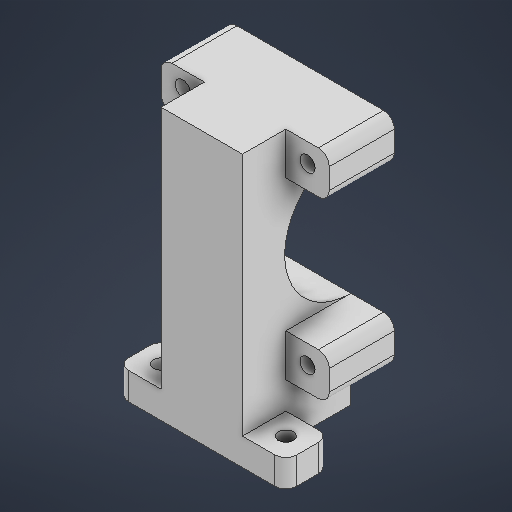
# Autodesk Inventor part: üst döner blok
Saved by Autodesk Inventor 2026.1 (Build 301233020, 233B)
## iProperties
Created: 2026-04-16
Part Number: üst döner blok
Material: Generic
Document SubType Name: Modeling
Designer: kadir
Density: 1 g/cm^3
Appearance: Default
Author: kadir
Autodesk Inventor part; units mm, degrees
ref_plane "YZ Plane" through (0, 0, 0) normal (1, 0, 0) x (0, 1, 0)
ref_plane "XZ Plane" through (0, 0, 0) normal (0, 1, 0) x (-1, 0, 0)
sketch "Sketch1" plane through (0, 0, 0) normal (0, 0, 1) x (1, 0, 0)
  line L0 (0, 0) -> (15, 0)
  line L1 (15, 0) -> (15, 50)
  line L2 (15, 50) -> (0, 50)
  line L3 (0, 50) -> (0, 0)
  dimension "d0" = 15
  dimension "d1" = 50
  constraints: 8 end point, 2 parallel, 1 horizontal, 1 perpendicular
  measures "d0" distance of L2.end L1.end
  measures "d1" distance of L1.end L0.end
extrude "Extrusion1" add sketch "Sketch1" along normal blind 20
sketch "Sketch2" plane through (15, 0, 0) normal (1, 0, 0) x (0, 0, -1)
  circle A0 centre (0, 30) radius 12.2
  line L0 (0, 50) -> (-20, 50) projected
  line L1 (0, 0) -> (0, 50) projected
  line L2 (0, 50) -> (0, 0)
  line L3 (-20, 0) -> (-20, 50) projected
  point P0 (0, 17.8)
  point P1 (0, 42.2)
  dimension "d4" = 24.4
  dimension "d5" = 20
  dimension "d6" = 20
  constraints: 2 end point, 1 centre point, 1 vertical
  measures "d4" diameter of A0
  measures "d5" distance from line of L0 A0.centre
  measures "d6" distance from line of L3 A0.centre
extrude "Extrusion2" cut sketch "Sketch2" against normal through all contours L1 A0 picked at (-4.6431, 33.0439)
sketch "Sketch3" plane through (15, 0, 20) normal (1, 0, 0) x (0, 0, -1)
  line L0 (20, 50) -> (0, 50) projected
  line L1 (20, 50) -> (8, 50)
  line L2 (8, 50) -> (8, 42.2)
  line L3 (8, 42.2) -> (20, 42.2)
  line L4 (20, 42.2) -> (20, 50)
  line L5 (-6.7049, 30) -> (32.7164, 30)
  line L6 (20, 10) -> (0, 10)
  line L7 (8, 10) -> (8, 17.8)
  line L8 (8, 17.8) -> (20, 17.8)
  line L9 (20, 17.8) -> (20, 10)
  point P0 (20, 0)
  dimension "d9" = 12
  dimension "d10" = 7.8
  dimension "d11" = 20
  constraints: 18 end point, 5 symmetric about line, 2 horizontal, 2 parallel, 1 perpendicular
  measures "d9" distance of L3.end L2.end
  measures "d10" distance of L2.end L1.end
  measures "d11" distance between parallel lines of L0 L5
extrude "Extrusion3" add sketch "Sketch3" along normal blind 8
sketch "Sketch4" plane through (0, 0, 0) normal (0, 0, -1) x (-1, 0, 0)
  circle A0 centre (-19, 46.5) radius 1.4
  line L0 (0, 50) -> (-23, 50) projected
  line L1 (-23, 42.2) -> (-23, 50) projected
  circle A1 centre (-19, 14.3) radius 1.4
  line L2 (-15, 17.8) -> (-23, 17.8) projected
  line L3 (-23, 10) -> (-23, 17.8) projected
  point P0 (0, 0)
  dimension "d14" = 2.8
  dimension "d15" = 3.5
  dimension "d16" = 4
  dimension "d17" = 2.8
  dimension "d18" = 3.5
  dimension "d43" = 4
  constraints: 2 centre point
  measures "d14" diameter of A0
  measures "d15" distance from line of L0 A0.centre
  measures "d16" distance from line of L1 A0.centre
  measures "d17" diameter of A1
  measures "d18" distance from line of L2 A1.centre
  measures "d43" distance from line of L3 A1.centre
extrude "Extrusion4" cut sketch "Sketch4" against normal through all
sketch "Sketch5" plane through (0, 0, 20) normal (-1, 0, 0) x (0, 0, 1)
  line L0 (-20, 42.2) -> (-20, 50) projected
  line L1 (-8, 42.2) -> (-20, 42.2) projected
  line L2 (-20, 50) -> (-8, 50)
  line L3 (-8, 50) -> (-8, 42.2)
  line L4 (-8, 42.2) -> (-20, 42.2)
  line L5 (-20, 42.2) -> (-20, 50)
  arc A0 (-20, 17.8) -> (-20, 42.2) centre (-20, 30) ccw projected
  line L6 (-8, 10) -> (-20, 10) projected
  line L7 (-20, 17.8) -> (-8, 17.8)
  line L8 (-8, 17.8) -> (-8, 10)
  line L9 (-8, 10) -> (-20, 10)
  line L10 (-20, 10) -> (-20, 17.8)
  point P0 (-20, 0)
  constraints: 16 end point, 4 parallel, 2 horizontal, 2 perpendicular
extrude "Extrusion5" add sketch "Sketch5" along normal blind 8
sketch "Sketch6" plane through (0, 0, 0) normal (0, 0, -1) x (-1, 0, 0)
  circle A0 centre (4, 47) radius 1.4
  line L0 (8, 50) -> (8, 42.2) projected
  line L1 (8, 50) -> (-23, 50) projected
  circle A1 centre (4, 14.8) radius 1.4
  line L2 (0, 17.8) -> (8, 17.8) projected
  line L3 (8, 17.8) -> (8, 10) projected
  point P0 (0, 0)
  point P1 (8, 46.1)
  dimension "d23" = 2.8
  dimension "d24" = 4
  dimension "d25" = 3
  dimension "d26" = 2.8
  dimension "d27" = 3
  dimension "d44" = 4
  constraints: 2 centre point, 1 midpoint
  measures "d23" diameter of A0
  measures "d24" horizontal distance of point (8, 46.1) A0.centre
  measures "d25" distance from line of L1 A0.centre
  measures "d26" diameter of A1
  measures "d27" distance from line of L2 A1.centre
  measures "d44" distance from line of L3 A1.centre
extrude "Extrusion6" cut sketch "Sketch6" against normal through all
ref_plane "Work Plane1" through (0, 0, 0) normal (0, -1, 0) x (1, 0, 0)
sketch "Sketch7" plane through (0, 0, 0) normal (0, -1, 0) x (1, 0, 0)
  line L0 (0, 0) -> (0, 20) projected
  line L1 (0, 20) -> (-8, 20)
  line L2 (-8, 20) -> (-8, 12)
  line L3 (-8, 12) -> (0, 12)
  line L4 (0, 12) -> (0, 20)
  line L5 (0, 0) -> (15, 0) projected
  line L6 (7.5, 0) -> (7.5, 20)
  line L7 (15, 20) -> (0, 20) projected
  circle A0 centre (-4, 16) radius 1.4
  line L8 (15, 0) -> (15, 20)
  line L9 (15, 20) -> (23, 20)
  line L10 (23, 20) -> (23, 12)
  line L11 (23, 12) -> (15, 12)
  circle A1 centre (19, 16) radius 1.4
  dimension "d30" = 8
  dimension "d31" = 8
  dimension "d32" = 2.8
  dimension "d41" = 4
  constraints: 18 end point, 4 symmetric about line, 2 centre point, 2 midpoint, 2 parallel, 1 horizontal, 1 perpendicular, 1 other
  measures "d30" distance of L3.end L2.end
  measures "d31" distance of L2.end L1.end
  measures "d32" diameter of A0
  measures "d41" distance from line of L0 A0.centre
extrude "Extrusion7" add sketch "Sketch7" against normal blind 5 contours L3 L2 L1 L0 | L8 L9 L10 L11
fillet "Fillet1" radius 2 2 edges at (23, 2.5, 20) (23, 2.5, 12)
fillet "Fillet2" radius 2 2 edges at (-8, 2.5, 12) (-8, 2.5, 20)
fillet "Fillet3" radius 2 2 edges at (23, 17.8, 6) (23, 10, 6)
fillet "Fillet4" radius 2 2 edges at (-8, 10, 6) (-8, 17.8, 6)
fillet "Fillet5" radius 2 2 edges at (-8, 50, 6) (-8, 42.2, 6)
fillet "Fillet6" radius 2 2 edges at (23, 50, 6) (23, 42.2, 6)
sketch "Sketch8" plane through (15, 10, 12) normal (0, 0, 1) x (1, 0, 0)
  point P0 (-15, -10)
sketch "Sketch9" plane through (0, 5, 0) normal (0, 1, 0) x (1, 0, 0)
  point P0 (0, 0)
sketch "Sketch10" plane through (15, 10, 12) normal (0, 0, 1) x (1, 0, 0)
  point P0 (-15, -10)
sketch "Sketch11" plane through (0, 42.2, 12) normal (0, 0, 1) x (1, 0, 0)
  point P0 (0, -42.2)
sketch "Sketch12" plane through (15, 42.2, 12) normal (0, 0, 1) x (1, 0, 0)
  point P0 (-15, -42.2)
sketch "Sketch13" plane through (0, 42.2, 12) normal (0, 0, 1) x (1, 0, 0)
  point P0 (0, -42.2)
body "Solid1"
